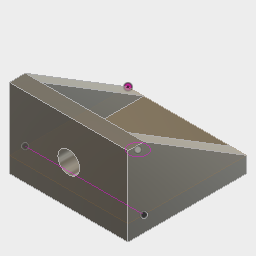
Power_Supply_Upper_Mount (Autodesk Fusion 360 design; units mm, degrees)
Autodesk Fusion 360 part; units mm, degrees
sketch "Sketch1" plane through (0, 0, 0) normal (0, 1, 0) x (1, 0, 0)
  line L0 (0, 0) -> (30, 0)
  line L1 (30, 0) -> (30, -30)
  line L2 (30, -30) -> (0, -30)
  line L3 (0, -30) -> (0, 0)
  dimension "d1" = 30
  dimension "d2" = 30
  measures "d1" distance of L0.start L0.end
  measures "d2" distance of L0.start L2.end
extrude "Extrude1" add sketch "Sketch1" along normal blind 4
sketch "Sketch2" plane through (0, 4, 0) normal (0, 1, 0) x (-1, 0, 0)
  line L0 (0, 30) -> (-30, 30)
  line L1 (-30, 30) -> (-30, 0)
  line L2 (-30, 0) -> (0, 0)
  line L3 (0, 0) -> (0, 30)
  circle A0 centre (-15, 12.5) radius 2.25
  line L4 (0, 26) -> (-30, 26)
  dimension "d5" = 4.5
  dimension "d6" = 12.5
  dimension "d7" = 15
  dimension "d23" = 4
  measures "d5" diameter of A0
  measures "d6" distance of L2 A0.centre
  measures "d7" distance of L3 A0.centre
  measures "d23" distance of L0 L4
hole "Hole1" at (15, 4, 12.5) direction (0, -1, 0) diameter 4.5 end through all
extrude "Extrude6" add sketch "Sketch2" along normal blind 16 contours L0 L1 L3 L4
sketch "Sketch7" plane through (0, 0, 30) normal (0, 0, 1) x (1, 0, 0)
  line L0 (0, 0) -> (30, 0)
  line L1 (30, 0) -> (30, 20)
  line L2 (30, 20) -> (0, 20)
  line L3 (0, 20) -> (0, 0)
  circle A0 centre (15, 10) radius 2.75
  dimension "d26" = 5.5
  dimension "d27" = 10
  measures "d26" diameter of A0
  measures "d27" distance of L2 A0.centre
extrude "Extrude7" cut sketch "Sketch7" against normal through all contours A0
sketch "Sketch8" plane through (0, 0, 0) normal (-1, 0, 0) x (0, 0, 1)
  line L0 (0, 0) -> (30, 0)
  line L1 (30, 0) -> (30, 20)
  line L2 (30, 20) -> (26, 20)
  line L3 (26, 20) -> (26, 4)
  line L4 (26, 4) -> (0, 4)
  line L5 (0, 4) -> (0, 0)
  line L6 (26, 20) -> (0, 4)
extrude "Extrude8" add sketch "Sketch8" against normal blind 4 contours L3 L4 L6
sketch "Sketch9" plane through (30, 0, 0) normal (1, 0, 0) x (0, 0, -1)
  line L0 (-30, 0) -> (0, 0)
  line L1 (0, 0) -> (0, 4)
  line L2 (0, 4) -> (-26, 4)
  line L3 (-26, 4) -> (-26, 20)
  line L4 (-26, 20) -> (-30, 20)
  line L5 (-30, 20) -> (-30, 0)
  line L6 (-26, 20) -> (0, 4)
extrude "Extrude9" add sketch "Sketch9" against normal blind 4 contours L2 L3 L6
